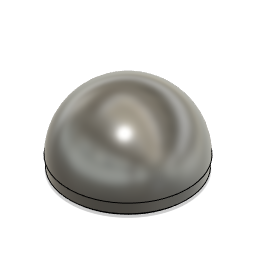
Ball_Topper (Autodesk Fusion 360 design; units mm, degrees)
Autodesk Fusion 360 part; units mm, degrees
sketch "Sketch1" plane through (0, 0, 0) normal (0, 0, 1) x (1, 0, 0)
  circle A0 centre (0, 0) radius 30
  line L0 (-14, -26.533) -> (-14, 0)
  line L1 (-14, 0) -> (14, 0)
  line L2 (14, 0) -> (14, -26.533)
  line L3 (-14, -6) -> (-29.3939, -6)
  line L4 (14, -6) -> (29.3939, -6)
  line L5 (-29.3939, -6) -> (-30, 0)
  line L6 (29.3939, -6) -> (30, 0)
  line L7 (14, 0) -> (30, 0) construction
  line L8 (-14, 0) -> (-30, 0) construction
  line L9 (0, 0) -> (0, 30)
  dimension "d1" = 60
  dimension "d2" = 28
  dimension "d7" = 6
  dimension "d8" = 6
  constraint coincident A0.centre L9.start
  constraint coincident A0 L0.start
  constraint vertical L0
  constraint perpendicular L0 L1
  constraint coincident A0 L2.end
  constraint perpendicular L1 L2
  constraint midpoint A0.centre L1
  constraint coincident L0 L3.start
  constraint coincident A0 L3.end
  constraint perpendicular L0 L3
  constraint coincident L2 L4.start
  constraint coincident A0 L4.end
  constraint perpendicular L2 L4
  constraint coincident A0 L5.end
  constraint coincident A0 L6.end
  constraint perpendicular L2 L7
  constraint perpendicular L0 L8
  constraint coincident A0 L9.end
  constraint perpendicular L1 L9
  measures "d1" diameter of A0
  measures "d2" distance of L0.end L1.end
  measures "d7" distance of L3 L8
  measures "d8" distance of L4 L7
revolve "Revolve1" add sketch "Sketch1" angle 360 about axis through (0, 0, 0) along (0, 1, 0) contours A0 L1 L2 L4 L6 L9
sketch "Sketch2" plane through (0, 0, 0) normal (0, -1, 0) x (1, 0, 0)
  circle A0 centre (0, 0) radius 14
  circle A1 centre (0, 0) radius 9
  dimension "d10" = 18
  constraint concentric A0 A1
  measures "d10" diameter of A1
extrude "Extrude1" cut sketch "Sketch2" against normal blind 3 contours A1
thread "Thread1" "ISO Metric profile 28.0 M28x2 6H" major diameter 28.2565 minor diameter 26.0224 pitch 2 angle 60 modelled right hand crest width 0.5434 on face at (13.9304, -4, 1.3939) crest through (13.0112, -0.5, 0)
sketch "Sketch3" plane through (0, 0, 0) normal (0, 0, 1) x (1, 0, 0)
  line L0 (9, 3) -> (-9, 3)
  line L1 (9, 0) -> (-9, 0)
  line L2 (9, 0) -> (7.6706, 3)
  line L3 (9, 3) -> (9, 0)
  line L4 (0, 0) -> (0, 3) construction
  dimension "d13" = 66.1
  constraint coincident L1.start L2.start
  constraint coincident L0 L2.end
  constraint coincident L0.start L3.start
  constraint coincident L4.start origin
  constraint midpoint L0 L4.end
  measures "d13" angle of L0 L2
revolve "Revolve2" add sketch "Sketch3" angle 360 about axis through (0, 0, 0) along (0, 1, 0)
sketch "Sketch4" plane through (0, 0, 0) normal (0, -1, 0) x (1, 0, 0)
  arc A0 (-9.8061, -8.5517) -> (9.8061, -8.5517) centre (0, 0) ccw
  spline S0 degree 3 poles (9.8061, -8.5517) (10.5142, -7.806) (11.1313, -6.9789) (12.1649, -5.1889) (12.5756, -4.2311) (13.3644, -1.5664) (13.5251, 0.1832) (13.1691, 3.6743) (12.6452, 5.381) (10.964, 8.5248) (9.8136, 9.9266) (7.0217, 12.2323) (5.4004, 13.1058) (3.6576, 13.6466) knots -2.761439 -2.761439 -2.761439 -2.761439 -2.452475 -2.452475 -2.140473 -2.140473 -1.617666 -1.617666 -1.08665 -1.08665 -0.547427 -0.547427 0 0 0 0
  arc A1 (3.6576, 13.6466) -> (-3.6576, 13.6466) centre (0, 0) ccw
  spline S1 degree 3 poles (-3.6576, 13.6466) (-4.7143, 13.3187) (-5.7287, 12.8678) (-7.6214, 11.7415) (-8.4942, 11.0722) (-10.5613, 9.057) (-11.589, 7.5703) (-13.0011, 4.3098) (-13.3814, 2.5718) (-13.4489, -0.9248) (-13.1459, -2.6494) (-11.901, -5.8577) (-10.9811, -7.3143) (-9.8061, -8.5517) knots -2.756672 -2.756672 -2.756672 -2.756672 -2.425266 -2.425266 -2.096892 -2.096892 -1.560377 -1.560377 -1.032054 -1.032054 -0.511928 -0.511928 0 0 0 0
  circle A2 centre (0, 0) radius 16
  line L0 (-13.2288, 9) -> (13.2288, 9)
  line L1 (9, 13.2288) -> (9, 9.5635)
  line L2 (9, 9.5635) -> (9, -13.2288)
  line L3 (13.2288, -9) -> (-13.2288, -9)
  line L4 (-9, -13.2288) -> (-9, 13.2288)
  circle A3 centre (0, 0) radius 9
  dimension "d22" = 32
  constraint horizontal L0
  constraint perpendicular L0 L1
  constraint coincident A2 L2.end
  constraint perpendicular L0 L2
  constraint coincident A2 L3.start
  constraint coincident A2 L3.end
  constraint perpendicular L2 L3
  constraint coincident A2 L4.start
  constraint coincident A2 L4.end
  constraint perpendicular L0 L4
  constraint tangent L0 A3
  constraint tangent L4 A3
  constraint tangent L3 A3
  constraint tangent L2 A3
  constraint coincident A2 L0.start
  constraint coincident A2 L1.start
  constraint coincident A2 L0.end
  constraint coincident A0.centre A1.centre
  measures "d22" diameter of A2
extrude "Extrude2" cut sketch "Sketch4" against normal blind 0.4 contours L3 L4 A3 | L0 L4 A3 | L2 L3 A3 | A3 | L0 L2 A3
extrude "Extrude3" cut sketch "Sketch4" against normal blind 0.2 contours A0 L2 L3 L4 | S0 A1 S1 L0 L1 L2 L4
chamfer "Chamfer3" distance 0.4 angle 45 1 edges at (-8.2257, 0.4, -3.1904)
chamfer "Chamfer4" distance 1 angle 45 1 edges at (-27.4047, -6, -10.6293)
equation "d1 = Diameter"
equation "Diameter = 60 mm" comment "35mm minimum"
named bodies: "Ball_Topper"
